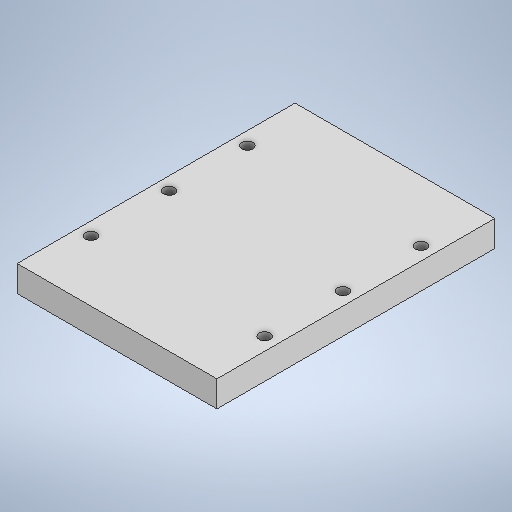
# Autodesk Inventor part: Part_Back
Saved by Autodesk Inventor 2025 (Build 290162010, 162A)
## iProperties
Created: 2024-07-05
Part Number: Part_Back
Material: Generic
Document SubType Name: Modeling
Designer: kani2
Density: 1 g/cm^3
Appearance: Default
Author: kani2
Autodesk Inventor part; units mm, degrees
ref_plane "YZ Plane" through (0, 0, 0) normal (1, 0, 0) x (0, 1, 0)
ref_plane "XZ Plane" through (0, 0, 0) normal (0, 1, 0) x (-1, 0, 0)
ref_plane "XY Plane" through (0, 0, 0) normal (0, 0, 1) x (1, 0, 0)
sketch "Sketch1" plane through (0, 0, 0) normal (0, 1, 0) x (-1, 0, 0)
  line L0 (73.025, 101.6) -> (-73.025, 101.6)
  line L1 (-73.025, 101.6) -> (-73.025, -101.6)
  line L2 (-73.025, -101.6) -> (73.025, -101.6)
  line L3 (73.025, -101.6) -> (73.025, 101.6)
  line L4 (73.025, 101.6) -> (-73.025, -101.6) construction
  line L5 (-73.025, 101.6) -> (73.025, -101.6) construction
  point P0 (0, 0)
  dimension "d0" = 146.05
  dimension "d1" = 203.2
  constraints: 12 end point, 2 midpoint, 2 parallel, 1 horizontal, 1 perpendicular
  measures "d0" distance of L2.end L1.end
  measures "d1" distance of L1.end L0.end
extrude "Extrusion1" add sketch "Sketch1" along normal blind 19.05
sketch "Sketch2" plane through (0, 19.05, 0) normal (0, 1, 0) x (1, 0, 0)
  circle A0 centre (-63.5, -57.15) radius 4.0894
  circle A1 centre (-63.5, 0) radius 4.0894
  circle A2 centre (-63.5, 57.15) radius 4.0894
  circle A3 centre (63.5, -57.15) radius 4.0894
  circle A4 centre (63.5, 0) radius 4.0894
  circle A5 centre (63.5, 57.15) radius 4.0894
  line L0 (-73.025, -101.6) -> (73.025, -101.6) projected
  line L1 (73.025, -101.6) -> (73.025, 101.6) projected
  line L2 (-73.025, 101.6) -> (-73.025, -101.6) projected
  point P0 (0, 0)
  dimension "d4" = 8.1788
  dimension "d5" = 8.1788
  dimension "d6" = 8.1788
  dimension "d7" = 8.1788
  dimension "d8" = 8.1788
  dimension "d9" = 8.1788
  dimension "d10" = 44.45
  dimension "d11" = 101.6
  dimension "d12" = 158.75
  dimension "d13" = 44.45
  dimension "d14" = 101.6
  dimension "d15" = 158.75
  dimension "d16" = 9.525
  dimension "d17" = 9.525
  dimension "d18" = 9.525
  dimension "d19" = 9.525
  dimension "d20" = 9.525
  dimension "d21" = 9.525
  constraints: 6 centre point
  measures "d4" diameter of A0
  measures "d5" diameter of A1
  measures "d6" diameter of A2
  measures "d7" diameter of A3
  measures "d8" diameter of A4
  measures "d9" diameter of A5
  measures "d10" distance from line of L0 A0.centre
  measures "d11" distance from line of L0 A1.centre
  measures "d12" distance from line of L0 A2.centre
  measures "d13" distance from line of L0 A3.centre
  measures "d14" distance from line of L0 A4.centre
  measures "d15" distance from line of L0 A5.centre
  measures "d16" distance from line of L1 A3.centre
  measures "d17" distance from line of L1 A4.centre
  measures "d18" distance from line of L1 A5.centre
  measures "d19" distance from line of L2 A0.centre
  measures "d20" distance from line of L2 A1.centre
  measures "d21" distance from line of L2 A2.centre
extrude "Extrusion2" cut sketch "Sketch2" against normal blind 19.05
body "Solid1"
